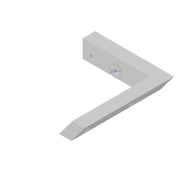
# Autodesk Inventor part: Delivery bin right angle connector
Saved by Autodesk Inventor 2018 (Build 220112000, 112)
## iProperties
Created: 2019-01-05
Part Number: Delivery bin right angle connector
Material: Generic
Document SubType Name: Modeling
Designer: ball
Density: 1 g/cm^3
Appearance: Default
Author: ball
Autodesk Inventor part; units mm, degrees
ref_plane "YZ Plane" through (0, 0, 0) normal (1, 0, 0) x (0, 1, 0)
ref_plane "XZ Plane" through (0, 0, 0) normal (0, 1, 0) x (-1, 0, 0)
ref_plane "Work Plane1" through (0, 0, 0) normal (0, 0, 1) x (1, 0, 0)
sketch "Sketch1" plane through (0, 0, 0) normal (0, 0, 1) x (1, 0, 0)
  line L0 (0, 14.859) -> (-322.453, 14.859) construction
  line L1 (-0.635, 0) -> (-321.818, 0) construction
  line L2 (0, 14.859) -> (0, 0.635) construction
  line L3 (2.54, 14.859) -> (2.54, 0) construction
  line L4 (2.54, 14.859) -> (17.399, 14.859) construction
  line L5 (2.54, 0) -> (-51.4985, 0)
  line L6 (13.7371, 14.859) -> (-30.6705, 14.859) construction
  circle A0 centre (-4.7625, 4.7625) radius 1.778 construction
  line L7 (-7.62, 0) -> (-7.62, 14.859) construction
  circle A1 centre (-24.3205, 4.7625) radius 1.778 construction
  circle A2 centre (-43.8785, 4.7625) radius 1.778 construction
  circle A3 centre (-24.3205, 4.7625) radius 1.9685
  circle A4 centre (-43.8785, 4.7625) radius 1.9685
  line L8 (-51.4985, 0) -> (-51.4985, 14.859)
  circle A5 centre (-24.3205, 4.7625) radius 4.8768 construction
  circle A6 centre (-43.8785, 4.7625) radius 4.8768 construction
  line L9 (13.7371, 14.859) -> (-51.4985, 14.859)
  line L10 (2.54, 0) -> (13.7371, 14.859)
  line L11 (2.54, 0) -> (21.1455, 0) construction
  point P0 (0, 0)
  dimension "d1" = 2.54
  dimension "d7" = 10.16
  dimension "d9" = 3.937
  dimension "d10" = 3.937
  dimension "d11" = 7.62
  dimension "d12" = 9.7536
  dimension "d13" = 9.7536
  dimension "d46" = 53
  constraints: 24 end point, 9 point on line, 7 centre point, 5 horizontal, 4 coincident, 2 collinear, 2 equal length, 2 perpendicular, 1 parallel, 1 vertical, 11 other
  measures "d1" distance between parallel lines of L2 L3
  measures "d7" distance between parallel lines of L7 L3
  measures "d9" diameter of A3
  measures "d10" diameter of A4
  measures "d11" distance from line of L8 A2.centre
  measures "d12" diameter of A5
  measures "d13" diameter of A6
  measures "d46" angle of L11 L10
extrude "Extrusion1" add sketch "Sketch1" along normal blind 10.16
sketch "Sketch2" plane through (0, 0, 10.16) normal (0, 0, 1) x (1, 0, 0)
  circle A0 centre (-24.3205, 4.7625) radius 1.9685 construction
  circle A1 centre (-43.8785, 4.7625) radius 1.9685 construction
  line L0 (13.7371, 14.859) -> (-51.4985, 14.859) projected
  line L1 (2.54, 0) -> (-7.62, 0)
  line L2 (3.5771, 14.859) -> (13.7371, 14.859)
  line L3 (2.54, 0) -> (13.7371, 14.859)
  line L4 (2.54, 0) -> (24.4372, 0) construction
  line L5 (-7.62, 0) -> (3.5771, 14.859)
  line L6 (-7.62, 0) -> (10.9855, 0) construction
  point P0 (0, 0)
  point P1 (2.54, 14.859)
  dimension "d35" = 53
  dimension "d45" = 53
  constraints: 12 end point, 3 horizontal, 1 equal length, 1 parallel
  measures "d35" angle of L4 L3
  measures "d45" angle of L6 L5
extrude "Extrusion2" add sketch "Sketch2" along normal blind 63.5 and the other way blind 10.16
sketch "Sketch4" plane through (0, 0, 10.16) normal (0, 0, 1) x (1, 0, 0)
  circle A0 centre (-24.3205, 4.7625) radius 1.9685 construction
  circle A1 centre (-24.3205, 4.7625) radius 4.8768 construction
  point P0 (0, 0)
  dimension "d25" = 9.7536
  constraints: 1 centre point, 1 coincident
  measures "d25" diameter of A1
sketch "Sketch7" plane through (13.7371, 14.859, 73.66) normal (0.7986, -0.6018, 0) x (0, 0, -1)
  line L0 (0, -18.6055) -> (0, 0) construction
  line L1 (0, -13.5255) -> (73.66, -13.5255) construction
  line L2 (73.66, -39.2597) -> (73.66, 0) construction
  line L3 (73.66, -18.6055) -> (0, -18.6055) construction
  circle A0 centre (10.16, -13.5255) radius 1.9685
  line L4 (73.66, -18.6055) -> (73.66, -51.1267) projected
  circle A1 centre (46.99, -13.5255) radius 1.9685
  point P0 (73.66, -20.1341)
  dimension "d38" = 5.08
  dimension "d39" = 3.937
  dimension "d40" = 63.5
  dimension "d41" = 3.937
  dimension "d42" = 26.67
  constraints: 3 point on line, 2 centre point, 2 end point, 1 horizontal
  measures "d38" distance between parallel lines of L3 L1
  measures "d39" diameter of A0
  measures "d40" distance from line of A0.centre L4
  measures "d41" diameter of A1
  measures "d42" distance from line of A1.centre L4
extrude "Extrusion5" cut sketch "Sketch7" against normal through all
body "Solid1"
